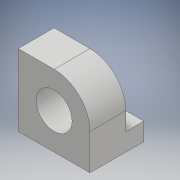
# Autodesk Inventor part: 20
Saved by Autodesk Inventor 2017 (Build 210142000, 142)
## iProperties
Part Number: 20
Material: 一般
Document SubType Name: Modeling
Designer: Brian
Density: 1 g/cm^3
Appearance: 預設
Author: Brian
Autodesk Inventor part; units mm, degrees
ref_plane "YZ Plane" through (0, 0, 0) normal (1, 0, 0) x (0, 1, 0)
ref_plane "XZ Plane" through (0, 0, 0) normal (0, 1, 0) x (-1, 0, 0)
ref_plane "XY Plane" through (0, 0, 0) normal (0, 0, 1) x (1, 0, 0)
sketch "草圖1" plane through (0, 0, 0) normal (0, 1, 0) x (-1, 0, 0)
  line L0 (0, 0) -> (-40, 0)
  line L1 (-40, 0) -> (-40, -40)
  line L2 (-40, -40) -> (0, -40)
  line L3 (0, -40) -> (0, 0)
  dimension "d0" = 40
  dimension "d1" = 40
  constraints: 8 end point, 2 parallel, 1 horizontal, 1 perpendicular
  measures "d0" distance of L1.end L2.end
  measures "d1" distance of L2.end L0.start
extrude "擠出1" add sketch "草圖1" along normal blind 20
sketch "草圖2" plane through (0, 0, -40) normal (-1, 0, 0) x (0, 0, 1)
  line L0 (40, 20) -> (30, 30)
  line L1 (30, 30) -> (20, 30)
  line L2 (20, 30) -> (10, 40)
  line L3 (10, 40) -> (0, 40)
  line L4 (40, 20) -> (0, 20) projected
  line L5 (0, 40) -> (0, 20)
  point P0 (40, 0)
  dimension "d4" = 20
  dimension "d5" = 10
  dimension "d6" = 10
  dimension "d7" = 10
  dimension "d8" = 10
  constraints: 10 end point, 1 horizontal, 1 parallel, 1 perpendicular
  measures "d4" distance of L3.end L4.end
  measures "d5" distance of L0.end L1.end
  measures "d6" horizontal distance of L1.end L2.end
  measures "d7" horizontal distance of L0.start L0.end
  measures "d8" distance between parallel lines of L4 L1
extrude "擠出2" add sketch "草圖2" against normal blind 10
sketch "草圖3" plane through (40, 0, -40) normal (0, 0, -1) x (-1, 0, 0)
  line L0 (40, 40) -> (30, 40) projected
  line L1 (30, 40) -> (20, 30)
  line L2 (20, 30) -> (20, 20)
  line L3 (30, 20) -> (0, 20) projected
  line L4 (30, 20) -> (30, 40)
  line L5 (30, 40) -> (30, 30) projected
  line L6 (20, 20) -> (30, 20)
  line L7 (0, 20) -> (10, 20)
  line L8 (10, 20) -> (10, 30)
  line L9 (10, 30) -> (0, 30)
  line L10 (0, 30) -> (0, 20)
  point P0 (40, 0)
  dimension "d11" = 10
  dimension "d12" = 10
  dimension "d13" = 10
  dimension "d14" = 10
  constraints: 16 end point, 3 point on line, 2 parallel, 1 collinear, 1 horizontal, 1 perpendicular, 1 vertical
  measures "d11" distance of L8.end L9.end
  measures "d12" distance of L7.end L8.end
  measures "d13" distance of L1.end L2.end
  measures "d14" horizontal distance of L0.end L1.end
extrude "擠出3" add sketch "草圖3" against normal blind 10
fillet "圓角1" radius 20 1 edges at (40, 10, 0)
hole "孔1" at (20, 0, -20) direction (0, 1, 0) diameter 20 depth 20 tip angle 118
